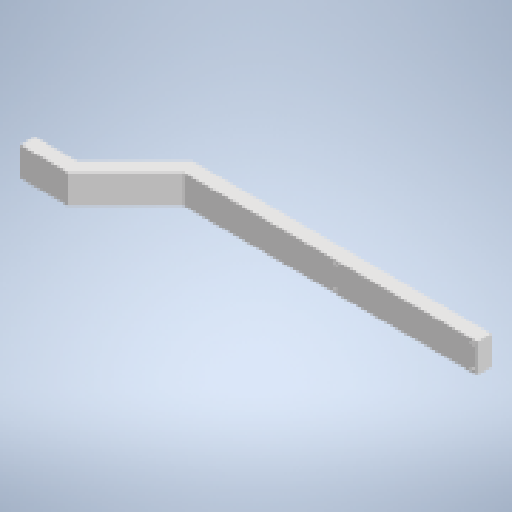
# Autodesk Inventor part: DOF2
Saved by Autodesk Inventor 2024 (Build 280153000, 153)
## iProperties
Created: 2024-10-15
Part Number: DOF2
Material: 一般
Document SubType Name: Modeling
Designer: jerry
Density: 1 g/cm^3
Appearance: 預設
Author: jerry
Autodesk Inventor part; units mm, degrees
ref_plane "YZ Plane" through (0, 0, 0) normal (1, 0, 0) x (0, 1, 0)
ref_plane "XZ Plane" through (0, 0, 0) normal (0, 1, 0) x (-1, 0, 0)
ref_plane "XY Plane" through (0, 0, 0) normal (0, 0, 1) x (1, 0, 0)
sketch "草圖1" plane through (0, 0, 0) normal (0, 0, 1) x (1, 0, 0)
  line L0 (-10, -30) -> (10, 30) construction
  line L1 (10, -30) -> (-10, 30) construction
  line L2 (10, 30) -> (-600, 30)
  line L3 (-600, 30) -> (-600, -30)
  line L4 (-600, -30) -> (10, -30)
  line L5 (10, -30) -> (10, 30)
  circle A0 centre (0, 22.5) radius 3
  circle A1 centre (0, -22.5) radius 3
  circle A2 centre (-285, 22.5) radius 3
  circle A3 centre (-285, -22.5) radius 3
  point P0 (0, 0)
  dimension "d0" = 20
  dimension "d1" = 60
  dimension "d2" = 610
  dimension "d4" = 6
  dimension "d5" = 6
  dimension "d8" = 6
  dimension "d9" = 6
  constraints: 12 end point, 4 centre point, 2 midpoint, 2 parallel, 1 horizontal, 1 perpendicular
  measures "d0" distance of L1.end L0.end
  measures "d1" distance of L0.end L1.start
  measures "d2" distance of L4.end L3.end
  measures "d4" diameter of A0
  measures "d5" diameter of A1
  measures "d8" diameter of A2
  measures "d9" diameter of A3
extrude "擠出1" add sketch "草圖1" along normal blind 30
sketch "草圖2" plane through (-600, -30, 0) normal (0, -1, 0) x (1, 0, 0)
  line L0 (0, 30) -> (-120.2082, 150.2082)
  line L1 (0, 30) -> (170, 30) construction
  line L2 (-120.2082, 150.2082) -> (-141.4214, 128.9949)
  line L3 (-141.4214, 128.9949) -> (-12.4264, 0)
  line L4 (0, 0) -> (610, 0) projected
  line L5 (-12.4264, 0) -> (0, 0)
  line L6 (0, 0) -> (0, 30)
  line L7 (-120.2082, 150.2082) -> (-220.2082, 150.2082)
  line L8 (-220.2082, 150.2082) -> (-220.2082, 120.2082)
  line L9 (-220.2082, 120.2082) -> (-132.6346, 120.2082)
  point P0 (600, 0)
  dimension "d13" = 170
  dimension "d14" = 135
  dimension "d15" = 30
  dimension "d16" = 100
  dimension "d17" = 30
  constraints: 18 end point, 4 perpendicular, 2 horizontal, 1 collinear, 1 equal length, 1 point on line
  measures "d13" distance of L0.start L0.end
  measures "d14" angle of L1 L0
  measures "d15" distance of L0.end L2.end
  measures "d16" distance of L0.end L7.end
  measures "d17" distance of L7.end L8.end
extrude "擠出2" add sketch "草圖2" against normal blind 60
